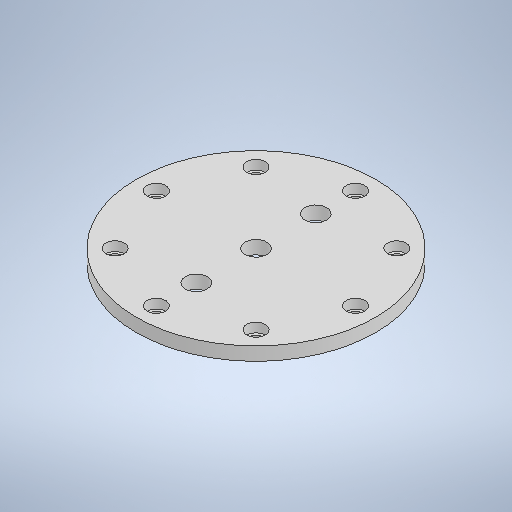
# Autodesk Inventor part: Part10
Saved by Autodesk Inventor 2025.2 (Build 292293000, 293)
## iProperties
Created: 2025-01-25
Part Number: Part10
Material: Generic
Document SubType Name: Modeling
Designer: caomi
Density: 1 g/cm^3
Appearance: Default
Author: caomi
Autodesk Inventor part; units mm, degrees
ref_plane "YZ Plane" through (0, 0, 0) normal (1, 0, 0) x (0, 1, 0)
ref_plane "XZ Plane" through (0, 0, 0) normal (0, 1, 0) x (-1, 0, 0)
ref_plane "XY Plane" through (0, 0, 0) normal (0, 0, 1) x (1, 0, 0)
sketch "Sketch1" plane through (0, 0, 0) normal (0, 1, 0) x (-1, 0, 0)
  circle A0 centre (0, 0) radius 45
  dimension "d0" = 90
  constraints: 1 centre point, 1 coincident
  measures "d0" diameter of A0
extrude "Extrusion1" add sketch "Sketch1" along normal blind 5
sketch "Sketch2" plane through (0, 5, 0) normal (0, 1, 0) x (1, 0, 0)
  point P0 (0, 0)
  point P1 (0, -37.5)
  dimension "d17" = 37.5
  constraints: 1 vertical alignment
  measures "d17" distance of point (0, -37.5) point (0, 0)
sketch "Sketch3" plane through (0, 5, 0) normal (0, 1, 0) x (1, 0, 0)
  circle A0 centre (0, -22.5) radius 4.1
  circle A1 centre (0, 22.5) radius 4.1
  line L0 (-27.2764, 0) -> (27.2764, 0) construction
  circle A2 centre (0, 0) radius 4.1
  dimension "d12" = 8.2
  dimension "d14" = 45
  constraints: 3 centre point, 2 coincident, 2 end point, 2 equal radius, 2 vertical alignment, 1 horizontal, 1 midpoint, 1 other
  measures "d12" diameter of A0
  measures "d14" distance of A0.centre A1.centre
extrude "Extrusion3" cut sketch "Sketch3" against normal up to surface (5 mm away)
hole "Hole1" at (0, 5, 37.5) direction (0, -1, 0) diameter 5 end through all counterbore diameter 7 counterbore depth 3.5
pattern_circular "Circular Pattern2" count 8 over 360 about axis through (0, 0, 0) along (0, 1, 0) of "Hole1"
body "Solid1"
